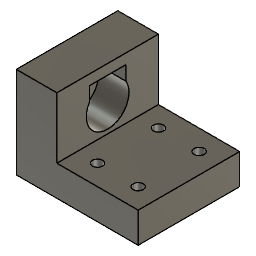
support_axe_x_proto2 (Autodesk Fusion 360 design; units mm, degrees)
Autodesk Fusion 360 part; units mm, degrees
note: some values were not read from the file. Set by a fixed rule: which sketch regions a step uses.
sketch "Esquisse1" plane through (0, 0, 0) normal (0, 1, 0) x (1, 0, 0)
sketch "Esquisse2" plane through (0, 0, 0) normal (0, 0, 1) x (1, 0, 0)
  line L0 (0, 0) -> (80, 0)
  line L1 (80, 0) -> (80, -50)
  line L2 (80, -50) -> (0, -50)
  line L3 (0, -50) -> (0, 0)
  constraint horizontal L0
  constraint vertical L1
  constraint horizontal L2
  constraint vertical L3
  constraint coincident L0.start L3.end
extrude "Extrusion1" add sketch "Esquisse2" along normal blind 10
sketch "Esquisse3" plane through (0, 0, 10) normal (0, 0, 1) x (-1, 0, 0)
  line L0 (0, 50) -> (-80, 50)
  line L1 (-80, 50) -> (-80, 0)
  line L2 (-80, 0) -> (0, 0)
  line L3 (0, 0) -> (0, 50)
  line L4 (0, 0) -> (-15, 0)
  line L5 (-15, 0) -> (-15, 50)
  line L6 (0, 50) -> (-15, 50)
  line L7 (0, 0) -> (0, 50)
  dimension "d3" = 15
  constraint coincident L2.end L3.start
  constraint perpendicular L3 L4
  constraint coincident L0 L5.end
  constraint perpendicular L0 L5
  constraint coincident L0.start L3.end
  measures "d3" distance of L2.end L4.end
sketch "Esquisse4" plane through (0, 0, 0) normal (0, 0, -1) x (1, 0, 0)
  line L0 (80, 50) -> (0, 50)
  line L1 (0, 50) -> (0, 0)
  line L2 (0, 0) -> (80, 0)
  line L3 (80, 0) -> (80, 50)
  line L4 (0, 50) -> (15, 50)
  line L5 (15, 50) -> (15, 0)
  line L6 (15, 0) -> (0, 0)
  line L7 (0, 0) -> (0, 50)
  dimension "d4" = 15
  constraint coincident L0.end L1.start
  constraint perpendicular L1 L4
  constraint coincident L2 L5.end
  constraint perpendicular L2 L5
  constraint perpendicular L1 L6
  constraint coincident L1.end L2.start
  measures "d4" distance of L0.end L4.end
extrude "Extrusion2" add sketch "Esquisse4" along normal blind 40 contours L0 L1 L2 L4 L5 L6 L7
sketch "Esquisse5" plane through (0, 0, 10) normal (0, 0, 1) x (-1, 0, 0)
  line L0 (-80, 0) -> (-80, 50)
  line L1 (-80, 25) -> (-15, 25)
  line L2 (-15, 25) -> (-20, 25)
  line L3 (-20, 25) -> (-20, 30)
  line L4 (-20, 30) -> (-20, 20)
  line L5 (-20, 20) -> (-33, 20)
  line L6 (-33, 20) -> (-33, 30)
  line L7 (-33, 30) -> (-20, 30)
  dimension "d7" = 65
  dimension "d8" = 13
  constraint vertical L0
  constraint midpoint L0 L1.start
  constraint perpendicular L0 L1
  constraint coincident L1 L2.end
  constraint perpendicular L2 L3
  constraint perpendicular L1 L4
  constraint perpendicular L4 L5
  constraint perpendicular L1 L6
  constraint perpendicular L3 L7
  measures "d7" distance of L1.start L1.end
  measures "d8" distance of L4.end L5.end
extrude "Extrusion3" cut sketch "Esquisse5" against normal blind 5
sketch "Esquisse6" plane through (15, 0, 0) normal (1, 0, 0) x (0, 1, 0)
  line L0 (0, 0) -> (-50, 0)
  line L1 (-50, 0) -> (-50, -40)
  line L2 (-50, -40) -> (0, -40)
  line L3 (0, -40) -> (0, 0)
  circle A0 centre (-40, -10) radius 2.5
  circle A1 centre (-10, -10) radius 2.5
  circle A2 centre (-40, -30) radius 2.5
  circle A3 centre (-10, -30) radius 2.5
  dimension "d11" = 5
  dimension "d12" = 5
  dimension "d13" = 5
  dimension "d14" = 5
  measures "d11" diameter of A0
  measures "d12" diameter of A1
  measures "d13" diameter of A2
  measures "d14" diameter of A3
hole "Perçage1" at (15, -40, -10) at (15, -10, -10) at (15, -10, -30) at (15, -40, -30) direction (-1, 0, 0) diameter 5 depth 15 tip angle 118
extrude "Extrusion4" cut 1 faces at (80, -16.6667, 3.3333) along direction (-1, 0, 0) blind 40
move_body "Déplacer1" bodies 1 to x (0, 0, 1) y (0, 1, 0) z (-1, 0, 0) at (22.9606, 0, -2.9606)
move_body "Déplacer2" bodies 1 to x (1, 0, 0) y (0, 1, 0) z (0, 0, 1) at (0, 0, 5)
move_body "Déplacer3" bodies 1 to x (1, 0, 0) y (0, 1, 0) z (0, 0, 1) at (0, 0, -2.5)
sketch "Esquisse7" plane through (0, 0, 0) normal (0, 1, 0) x (-1, 0, 0)
  line L0 (-12.9606, 39.5394) -> (-22.9606, 39.5394)
  line L1 (-22.9606, 39.5394) -> (-22.9606, 14.5394)
  line L2 (-22.9606, 14.5394) -> (-62.9606, 14.5394)
  line L3 (-62.9606, 14.5394) -> (-62.9606, -0.4606)
  line L4 (-62.9606, -0.4606) -> (-12.9606, -0.4606)
  line L5 (-12.9606, -0.4606) -> (-12.9606, 39.5394)
  line L6 (-12.9606, -0.4606) -> (-12.9606, 0)
  constraint coincident L4.end L5.start
  constraint coincident L5 L6.end
move_body "Déplacer4" bodies 1 to x (1, 0, 0) y (0, 1, 0) z (0, 0, 1) at (0, 0, 0.46)
extrude "Extrusion5" add 1 faces at (17.9606, -23.3333, 28.6661) along direction (-1, 0, 0) blind 5
extrude "Extrusion6" add 1 faces at (19.6272, -16.6667, 39.9994) along direction (0, 0, 1) blind 5
sketch "Esquisse8" plane through (22.9606, 0, 0) normal (1, 0, 0) x (0, 1, 0)
  line L0 (-50, 44.9994) -> (-50, 14.9994)
  line L1 (-50, 14.9994) -> (0, 14.9994)
  line L2 (0, 14.9994) -> (0, 44.9994)
  line L3 (0, 44.9994) -> (-50, 44.9994)
  line L4 (-50, 44.9994) -> (-25, 44.9994)
  line L5 (-25, 44.9994) -> (-25, 14.9994)
  circle A0 centre (-25, 27.5) radius 10.5
  line L6 (-25, 38) -> (-25, 40)
  line L7 (-25, 40) -> (-16, 40)
  line L8 (-16, 40) -> (-16, 32.9083)
  line L9 (-25, 40) -> (-34, 40)
  line L10 (-34, 40) -> (-34, 32.9083)
  constraint coincident L0.start L3.end
  constraint midpoint L3 L4.end
  constraint midpoint L1 L5.end
  constraint coincident L5 L6.start
  constraint coincident A0 L6.start
  constraint coincident L5 L6.end
  constraint perpendicular L6 L7
  constraint coincident A0 L8.end
  constraint perpendicular L7 L8
  constraint perpendicular L5 L9
  constraint coincident A0 L10.end
  constraint perpendicular L9 L10
extrude "Extrusion7" add 1 faces at (12.9606, -33.3333, 29.9994) along direction (-1, 0, 0) blind 10
extrude "Extrusion8" cut sketch "Esquisse8" against normal blind 15 contours L5 A0 L6 L7 L8 | L5 A0 L6 L9 L10 | L5 A0 | L5 A0
